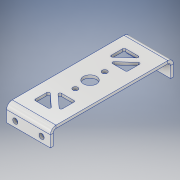
# Autodesk Inventor part: fc17-036
Saved by Autodesk Inventor 2017.1 (Build 211199000, 199)
## iProperties
Category: Controls
Company: Autodesk Inc.
Created: 2016-12-15
Part Number: fc17-036
Material: Aluminum 6061
Document SubType Name: Sheet Metal
Designer: Autodesk Inc.
Density: 2.7 g/cm^3
Sheet Metal Rule: Default
Appearance: Aluminum - Flat
Catalog Web Link: http://files.andymark.com/Camera-Pan-Tilt-Assembly.pdf
Vendor: ebm papst
Author: Autodesk Inc.
Keywords: FIRSTChoice
Autodesk Inventor part; units mm, degrees
ref_plane "YZ Plane" through (0, 0, 0) normal (1, 0, 0) x (0, 1, 0)
ref_plane "XZ Plane" through (0, 0, 0) normal (0, 1, 0) x (-1, 0, 0)
ref_plane "XY Plane" through (0, 0, 0) normal (0, 0, 1) x (1, 0, 0)
sketch "Sketch1" plane through (0, 0, 0) normal (0, 1, 0) x (-1, 0, 0)
  line L0 (0, 0) -> (25.4, 0)
  line L1 (25.4, 0) -> (25.4, -71.3232)
  line L2 (25.4, -71.3232) -> (0, -71.3232)
  line L3 (0, -71.3232) -> (0, 0)
  dimension "d0" = 25.4
  dimension "d1" = 71.3232
  measures "d0" distance of L1.end L2.end
  measures "d1" distance of L0.end L1.end
extrude "Plate1" add sketch "Sketch1" against normal blind 1.6281
sketch "Sketch2" plane through (-25.4, 0, -1.6281) normal (0, 0, 1) x (1, 0, 0)
  line L0 (25.4, 0) -> (0, 0)
  line L1 (0, 0) -> (0, -9.8298)
  line L2 (0, -9.8298) -> (25.4, -9.8298)
  line L3 (25.4, -9.8298) -> (25.4, 0)
  constraints: 6 end point, 1 horizontal, 1 perpendicular, 1 vertical
edge flange "Flange1" height 9.8298 angle 90 thickness 1.6281 bend radius 1.6281 thickness toward (0, 0, 1) relief straight relief width 1.6281 relief depth 0.8141 corner gap 1.6281 corner form 0 edges at (-12.7, -1.6281, 0) (-12.7, -1.6281, -71.3232) wall of the first edge with corners at (0, 0, -1.6281) (-25.4, 0, -1.6281) (-25.4, -9.8298, -1.6281) (0, -9.8298, -1.6281)
bend "Bend1"
corner "Corner1"
sketch "Sketch3" plane through (0, 0, 0) normal (0, 1, 0) x (1, 0, 0)
  circle A0 centre (-12.6937, 27.1526) radius 1.4351
  circle A1 centre (-12.6937, 44.1706) radius 1.4732
  line L0 (0.0063, 68.3192) -> (-25.3937, 68.3192)
  line L1 (-25.3937, 3.1844) -> (-25.3937, 68.3192)
  line L2 (-25.3937, 3.1844) -> (0.0063, 3.1844)
  line L3 (0.0063, 68.3192) -> (0.0063, 3.1844)
  line L4 (-14.4875, 50.5206) -> (-7.1374, 50.5206)
  line L5 (-6.3437, 51.3143) -> (-6.3437, 57.9882)
  line L6 (-7.671, 58.5758) -> (-15.0211, 51.902)
  line L7 (-10.3446, 60.4168) -> (-17.7227, 53.7176)
  line L8 (-19.05, 54.3052) -> (-19.05, 61.0044)
  line L9 (-18.2563, 61.7982) -> (-10.8781, 61.7982)
  line L10 (-14.4717, 20.8026) -> (-7.1374, 20.8026)
  line L11 (-6.3437, 20.0088) -> (-6.3437, 13.335)
  line L12 (-7.6716, 12.7479) -> (-15.0059, 19.4218)
  line L13 (-10.9157, 9.525) -> (-18.2563, 9.525)
  line L14 (-19.05, 10.3188) -> (-19.05, 17.018)
  line L15 (-17.7212, 17.6043) -> (-10.3806, 10.905)
  arc A2 (-6.3437, 57.9882) -> (-7.671, 58.5758) centre (-7.1374, 57.9882) ccw
  arc A3 (-7.1374, 50.5206) -> (-6.3437, 51.3143) centre (-7.1374, 51.3143) ccw
  arc A4 (-15.0211, 51.902) -> (-14.4875, 50.5206) centre (-14.4875, 51.3144) ccw
  arc A5 (-19.05, 54.3052) -> (-17.7227, 53.7176) centre (-18.2563, 54.3052) ccw
  arc A6 (-18.2563, 61.7982) -> (-19.05, 61.0044) centre (-18.2563, 61.0044) ccw
  arc A7 (-10.3446, 60.4168) -> (-10.8781, 61.7982) centre (-10.8781, 61.0044) ccw
  arc A8 (-6.3437, 20.0088) -> (-7.1374, 20.8026) centre (-7.1374, 20.0088) ccw
  arc A9 (-7.6716, 12.7479) -> (-6.3437, 13.335) centre (-7.1374, 13.335) ccw
  arc A10 (-14.4717, 20.8026) -> (-15.0059, 19.4218) centre (-14.4717, 20.0089) ccw
  arc A11 (-10.9157, 9.525) -> (-10.3806, 10.905) centre (-10.9157, 10.3188) ccw
  arc A12 (-19.05, 10.3188) -> (-18.2563, 9.525) centre (-18.2563, 10.3188) ccw
  arc A13 (-17.7212, 17.6043) -> (-19.05, 17.018) centre (-18.2562, 17.018) ccw
  line L16 (0, 0) -> (-25.4, 0) projected
  circle A14 centre (-12.6937, 35.6616) radius 3.81
  dimension "d28" = 0.7937
  dimension "d29" = 9.525
  dimension "d30" = 20.8026
  dimension "d32" = 17.018
  dimension "d34" = 27.1526
  dimension "d35" = 44.1706
  dimension "d36" = 50.5206
  dimension "d37" = 61.7982
  dimension "d38" = 13.335
  dimension "d39" = 6.35
  dimension "d40" = 35.6616
  dimension "d41" = 54.3052
  dimension "d42" = 57.9882
  dimension "d43" = 7.1437
  dimension "d44" = 10.922
  dimension "d45" = 12.7
  dimension "d46" = 14.478
  dimension "d47" = 18.2626
  dimension "d48" = 19.0563
  dimension "d49" = 25.4
  dimension "d50" = 7.62
  constraints: 32 end point, 24 point on circle, 24 tangent, 15 centre point, 11 equal radius, 5 vertical alignment, 3 parallel, 2 collinear, 2 perpendicular, 1 coincident
  measures "d28" radius of A2
  measures "d29" distance between parallel lines of L13 L16
  measures "d30" distance between parallel lines of L16 L10
  measures "d32" distance from line of A13.centre L16
  measures "d34" distance from line of A0.centre L16
  measures "d35" distance from line of A1.centre L16
  measures "d36" distance between parallel lines of L4 L16
  measures "d37" distance between parallel lines of L9 L16
  measures "d38" distance from line of A9.centre L16
  measures "d39" distance between parallel lines of L11 L3
  measures "d40" distance from line of point (-12.694, 35.662) L16
  measures "d41" distance from line of A5.centre L16
  measures "d42" distance from line of A2.centre L16
  measures "d43" distance from line of A9.centre L3
  measures "d44" distance from line of A11.centre L3
  measures "d45" distance from line of point (-12.694, 35.662) L3
  measures "d46" distance from line of A10.centre L3
  measures "d47" distance from line of A13.centre L3
  measures "d48" distance between parallel lines of L14 L3
  measures "d49" distance between parallel lines of L1 L3
  measures "d50" diameter of A14
extrude "Cut1" cut sketch "Sketch3" against normal blind 1.6281 contours A0 | A1 | A4 L6 A2 L5 A3 L4 | L7 A5 L8 A6 L9 A7 | L10 A8 L11 A9 L12 A10 | L13 A12 L14 A13 L15 A11 | A14
sketch "Sketch4" plane through (-25.4, -9.8298, 0) normal (0, 0, 1) x (1, 0, 0)
  line L0 (0, 0) -> (0, 6.5735) projected
  line L1 (0, 9.8298) -> (25.4, 9.8298) projected
  point P0 (5.08, 3.3274)
  point P1 (20.32, 3.3274)
  dimension "d53" = 5.08
  dimension "d54" = 20.32
  dimension "d55" = 6.5024
  constraints: 1 horizontal alignment
  measures "d53" distance from line of point (5.08, 3.327) L0
  measures "d54" distance from line of point (20.32, 3.327) L0
  measures "d55" distance from line of point (5.08, 3.327) L1
hole "Hole1" at (-20.32, -6.5024, 0) at (-5.08, -6.5024, 0) direction (0, 0, -1) diameter 2.9464 end up to surface
equation "\"d51\" = Thickness"
equation "\"d61\" = Thickness"
equation "\"d3\" = BendReliefWidth"
equation "\"d4\" = BendReliefDepth"
equation "\"d5\" = MinimumRemnant"
equation "\"d6\" = BendRadius"
equation "\"d9\" = BendRadius"
equation "\"d10\" = CornerReliefSize"
equation "\"d11\" = GapSize"
equation "\"d12\" = JacobiRadiusSize"
equation "\"BendRadius\" = Thickness"
equation "\"BendReliefWidth\" = Thickness"
equation "\"BendReliefDepth\" = 0.5 * Thickness"
equation "\"CornerReliefSize\" = 4 * Thickness"
equation "\"MinimumRemnant\" = 2 * Thickness"
equation "\"TransitionRadius\" = BendRadius"
equation "\"JacobiRadiusSize\" = BendRadius"
equation "\"GapSize\" = Thickness"
equation "\"d2\" = BendRadius"
equation "\"Thickness\" = 1.62814"
body "Solid1"
